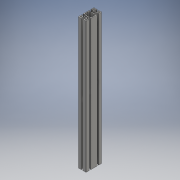
# Autodesk Inventor part: 240614_day3060_500
Saved by Autodesk Inventor 2016 (Build 200138000, 138)
## iProperties
Created: 2024-06-14
Part Number: 240614_day3060_500
Material: 일반
Document SubType Name: Modeling
Designer: pc
Density: 1 g/cm^3
Appearance: 기본값
Author: pc
Autodesk Inventor part; units mm, degrees
ref_plane "YZ Plane" through (0, 0, 0) normal (1, 0, 0) x (0, 1, 0)
ref_plane "XZ Plane" through (0, 0, 0) normal (0, 1, 0) x (-1, 0, 0)
ref_plane "XY Plane" through (0, 0, 0) normal (0, 0, 1) x (1, 0, 0)
sketch "스케치1" plane through (0, 0, 0) normal (0, 0, 1) x (1, 0, 0)
  line L0 (-12.2024, 9.85) -> (-6.681, 9.85)
  arc A0 (-6.681, 9.85) -> (-6.4593, 9.9479) centre (-6.681, 10.15) ccw
  arc A1 (-6.4593, 9.9479) -> (-4.5203, 14.4821) centre (-12.0024, 15) ccw
  line L1 (-4.5203, 14.4821) -> (-4.0024, 15)
  line L2 (-4.0024, 15) -> (-4.5203, 15.5179)
  arc A2 (-4.5203, 15.5179) -> (-6.4593, 20.0521) centre (-12.0024, 15) ccw
  arc A3 (-6.4593, 20.0521) -> (-6.681, 20.15) centre (-6.681, 19.85) ccw
  line L3 (-6.681, 20.15) -> (-12.2024, 20.15)
  arc A4 (-12.2024, 20.15) -> (-12.5024, 19.85) centre (-12.2024, 19.85) ccw
  line L4 (-12.5024, 19.85) -> (-12.5024, 18.45)
  arc A5 (-12.8024, 18.15) -> (-12.5024, 18.45) centre (-12.8024, 18.45) ccw
  line L5 (-12.8024, 18.15) -> (-15.0024, 18.15)
  line L6 (-15.0024, 18.15) -> (-15.0024, 28.9756)
  arc A6 (-14.0024, 29.9756) -> (-15.0024, 28.9756) centre (-14.0024, 28.9756) ccw
  line L7 (-14.0024, 29.9756) -> (-3.1524, 29.9756)
  line L8 (-3.1524, 29.9756) -> (-3.1524, 27.8)
  arc A7 (-3.4524, 27.5) -> (-3.1524, 27.8) centre (-3.4524, 27.8) ccw
  line L9 (-3.4524, 27.5) -> (-4.8524, 27.5)
  arc A8 (-4.8524, 27.5) -> (-5.1524, 27.2) centre (-4.8524, 27.2) ccw
  line L10 (-5.1524, 27.2) -> (-5.1524, 21.6786)
  arc A9 (-5.1524, 21.6786) -> (-5.0545, 21.4569) centre (-4.8524, 21.6786) ccw
  arc A10 (-5.0545, 21.4569) -> (-0.5203, 19.5179) centre (-0.0024, 27) ccw
  line L11 (-0.5203, 19.5179) -> (-0.0024, 19)
  line L12 (-0.0024, 19) -> (0.5155, 19.5179)
  arc A11 (0.5155, 19.5179) -> (5.0497, 21.4569) centre (-0.0024, 27) ccw
  arc A12 (5.0497, 21.4569) -> (5.1476, 21.6786) centre (4.8476, 21.6786) ccw
  line L13 (5.1476, 21.6786) -> (5.1476, 27.2)
  arc A13 (5.1476, 27.2) -> (4.8476, 27.5) centre (4.8476, 27.2) ccw
  line L14 (4.8476, 27.5) -> (3.4476, 27.5)
  arc A14 (3.1476, 27.8) -> (3.4476, 27.5) centre (3.4476, 27.8) ccw
  line L15 (3.1476, 27.8) -> (3.1476, 29.9756)
  line L16 (3.1476, 29.9756) -> (13.9976, 29.9756)
  arc A15 (14.9976, 28.9756) -> (13.9976, 29.9756) centre (13.9976, 28.9756) ccw
  line L17 (14.9976, 28.9756) -> (14.9976, 18.15)
  line L18 (14.9976, 18.15) -> (12.7976, 18.15)
  arc A16 (12.4976, 18.45) -> (12.7976, 18.15) centre (12.7976, 18.45) ccw
  line L19 (12.4976, 18.45) -> (12.4976, 19.85)
  arc A17 (12.4976, 19.85) -> (12.1976, 20.15) centre (12.1976, 19.85) ccw
  line L20 (12.1976, 20.15) -> (6.6762, 20.15)
  arc A18 (6.6762, 20.15) -> (6.4544, 20.0521) centre (6.6762, 19.85) ccw
  arc A19 (6.4544, 20.0521) -> (4.5155, 15.5179) centre (11.9976, 15) ccw
  line L21 (4.5155, 15.5179) -> (3.9976, 15)
  line L22 (3.9976, 15) -> (4.5155, 14.4821)
  arc A20 (4.5155, 14.4821) -> (6.4544, 9.9479) centre (11.9976, 15) ccw
  arc A21 (6.4544, 9.9479) -> (6.6762, 9.85) centre (6.6762, 10.15) ccw
  line L23 (6.6762, 9.85) -> (12.1976, 9.85)
  arc A22 (12.1976, 9.85) -> (12.4976, 10.15) centre (12.1976, 10.15) ccw
  line L24 (12.4976, 10.15) -> (12.4976, 11.55)
  arc A23 (12.7976, 11.85) -> (12.4976, 11.55) centre (12.7976, 11.55) ccw
  line L25 (12.7976, 11.85) -> (14.9976, 11.85)
  line L26 (14.9976, 11.85) -> (14.9976, -11.85)
  line L27 (14.9976, -11.85) -> (12.7976, -11.85)
  arc A24 (12.4976, -11.55) -> (12.7976, -11.85) centre (12.7976, -11.55) ccw
  line L28 (12.4976, -11.55) -> (12.4976, -10.15)
  arc A25 (12.4976, -10.15) -> (12.1976, -9.85) centre (12.1976, -10.15) ccw
  line L29 (12.1976, -9.85) -> (6.6762, -9.85)
  arc A26 (6.6762, -9.85) -> (6.4544, -9.9479) centre (6.6762, -10.15) ccw
  arc A27 (6.4544, -9.9479) -> (4.5155, -14.4821) centre (11.9976, -15) ccw
  line L30 (4.5155, -14.4821) -> (3.9976, -15)
  line L31 (3.9976, -15) -> (4.5155, -15.5179)
  arc A28 (4.5155, -15.5179) -> (6.4544, -20.0521) centre (11.9976, -15) ccw
  arc A29 (6.4544, -20.0521) -> (6.6762, -20.15) centre (6.6762, -19.85) ccw
  line L32 (6.6762, -20.15) -> (12.1976, -20.15)
  arc A30 (12.1976, -20.15) -> (12.4976, -19.85) centre (12.1976, -19.85) ccw
  line L33 (12.4976, -19.85) -> (12.4976, -18.45)
  arc A31 (12.7976, -18.15) -> (12.4976, -18.45) centre (12.7976, -18.45) ccw
  line L34 (12.7976, -18.15) -> (14.9976, -18.15)
  line L35 (14.9976, -18.15) -> (14.9976, -29.0244)
  arc A32 (13.9976, -30.0244) -> (14.9976, -29.0244) centre (13.9976, -29.0244) ccw
  line L36 (13.9976, -30.0244) -> (3.1476, -30.0244)
  line L37 (3.1476, -30.0244) -> (3.1476, -27.8)
  arc A33 (3.4476, -27.5) -> (3.1476, -27.8) centre (3.4476, -27.8) ccw
  line L38 (3.4476, -27.5) -> (4.8476, -27.5)
  arc A34 (4.8476, -27.5) -> (5.1476, -27.2) centre (4.8476, -27.2) ccw
  line L39 (5.1476, -27.2) -> (5.1476, -21.6786)
  arc A35 (5.1476, -21.6786) -> (5.0497, -21.4569) centre (4.8476, -21.6786) ccw
  arc A36 (5.0497, -21.4569) -> (0.5155, -19.5179) centre (-0.0024, -27) ccw
  line L40 (0.5155, -19.5179) -> (-0.0024, -19)
  line L41 (-0.0024, -19) -> (-0.5203, -19.5179)
  arc A37 (-0.5203, -19.5179) -> (-5.0545, -21.4569) centre (-0.0024, -27) ccw
  arc A38 (-5.0545, -21.4569) -> (-5.1524, -21.6786) centre (-4.8524, -21.6786) ccw
  line L42 (-5.1524, -21.6786) -> (-5.1524, -27.2)
  arc A39 (-5.1524, -27.2) -> (-4.8524, -27.5) centre (-4.8524, -27.2) ccw
  line L43 (-4.8524, -27.5) -> (-3.4524, -27.5)
  arc A40 (-3.1524, -27.8) -> (-3.4524, -27.5) centre (-3.4524, -27.8) ccw
  line L44 (-3.1524, -27.8) -> (-3.1524, -30.0244)
  line L45 (-3.1524, -30.0244) -> (-14.0024, -30.0244)
  arc A41 (-15.0024, -29.0244) -> (-14.0024, -30.0244) centre (-14.0024, -29.0244) ccw
  line L46 (-15.0024, -29.0244) -> (-15.0024, -18.15)
  line L47 (-15.0024, -18.15) -> (-12.8024, -18.15)
  arc A42 (-12.5024, -18.45) -> (-12.8024, -18.15) centre (-12.8024, -18.45) ccw
  line L48 (-12.5024, -18.45) -> (-12.5024, -19.85)
  arc A43 (-12.5024, -19.85) -> (-12.2024, -20.15) centre (-12.2024, -19.85) ccw
  line L49 (-12.2024, -20.15) -> (-6.681, -20.15)
  arc A44 (-6.681, -20.15) -> (-6.4593, -20.0521) centre (-6.681, -19.85) ccw
  arc A45 (-6.4593, -20.0521) -> (-4.5203, -15.5179) centre (-12.0024, -15) ccw
  line L50 (-4.5203, -15.5179) -> (-4.0024, -15)
  line L51 (-4.0024, -15) -> (-4.5203, -14.4821)
  arc A46 (-4.5203, -14.4821) -> (-6.4593, -9.9479) centre (-12.0024, -15) ccw
  arc A47 (-6.4593, -9.9479) -> (-6.681, -9.85) centre (-6.681, -10.15) ccw
  line L52 (-6.681, -9.85) -> (-12.2024, -9.85)
  arc A48 (-12.2024, -9.85) -> (-12.5024, -10.15) centre (-12.2024, -10.15) ccw
  line L53 (-12.5024, -10.15) -> (-12.5024, -11.55)
  arc A49 (-12.8024, -11.85) -> (-12.5024, -11.55) centre (-12.8024, -11.55) ccw
  line L54 (-12.8024, -11.85) -> (-15.0024, -11.85)
  line L55 (-15.0024, -11.85) -> (-15.0024, 11.85)
  line L56 (-15.0024, 11.85) -> (-12.8024, 11.85)
  arc A50 (-12.5024, 11.55) -> (-12.8024, 11.85) centre (-12.8024, 11.55) ccw
  line L57 (-12.5024, 11.55) -> (-12.5024, 10.15)
  arc A51 (-12.5024, 10.15) -> (-12.2024, 9.85) centre (-12.2024, 10.15) ccw
  arc A52 (-2.2146, 16.16) -> (-2.2146, 13.84) centre (0, 15) ccw
  line L58 (-2.2146, 13.84) -> (-2.79, 13.2645)
  arc A53 (-2.79, 13.2645) -> (-2.79, 12.8403) centre (-2.5779, 13.0524) ccw
  line L59 (-2.79, 12.8403) -> (-2.1597, 12.21)
  arc A54 (-2.1597, 12.21) -> (-1.7355, 12.21) centre (-1.9476, 12.4221) ccw
  line L60 (-1.7355, 12.21) -> (-1.16, 12.7854)
  arc A55 (-1.16, 12.7854) -> (1.16, 12.7854) centre (0, 15) ccw
  line L61 (1.16, 12.7854) -> (1.7355, 12.21)
  arc A56 (1.7355, 12.21) -> (2.1597, 12.21) centre (1.9476, 12.4221) ccw
  line L62 (2.1597, 12.21) -> (2.79, 12.8403)
  arc A57 (2.79, 12.8403) -> (2.79, 13.2645) centre (2.5779, 13.0524) ccw
  line L63 (2.79, 13.2645) -> (2.2146, 13.84)
  arc A58 (2.2146, 13.84) -> (2.2146, 16.16) centre (0, 15) ccw
  line L64 (2.2146, 16.16) -> (2.79, 16.7355)
  arc A59 (2.79, 16.7355) -> (2.79, 17.1597) centre (2.5779, 16.9476) ccw
  line L65 (2.79, 17.1597) -> (2.1597, 17.79)
  arc A60 (2.1597, 17.79) -> (1.7355, 17.79) centre (1.9476, 17.5779) ccw
  line L66 (1.7355, 17.79) -> (1.16, 17.2146)
  arc A61 (1.16, 17.2146) -> (-1.16, 17.2146) centre (0, 15) ccw
  line L67 (-1.16, 17.2146) -> (-1.7355, 17.79)
  arc A62 (-1.7355, 17.79) -> (-2.1597, 17.79) centre (-1.9476, 17.5779) ccw
  line L68 (-2.1597, 17.79) -> (-2.79, 17.1597)
  arc A63 (-2.79, 17.1597) -> (-2.79, 16.7355) centre (-2.5779, 16.9476) ccw
  line L69 (-2.79, 16.7355) -> (-2.2146, 16.16)
  line L70 (-1.16, -12.7854) -> (-1.7355, -12.21)
  arc A64 (-1.7355, -12.21) -> (-2.1597, -12.21) centre (-1.9476, -12.4221) ccw
  line L71 (-2.1597, -12.21) -> (-2.79, -12.8403)
  arc A65 (-2.79, -12.8403) -> (-2.79, -13.2645) centre (-2.5779, -13.0524) ccw
  line L72 (-2.79, -13.2645) -> (-2.2146, -13.84)
  arc A66 (-2.2146, -13.84) -> (-2.2146, -16.16) centre (0, -15) ccw
  line L73 (-2.2146, -16.16) -> (-2.79, -16.7355)
  arc A67 (-2.79, -16.7355) -> (-2.79, -17.1597) centre (-2.5779, -16.9476) ccw
  line L74 (-2.79, -17.1597) -> (-2.1597, -17.79)
  arc A68 (-2.1597, -17.79) -> (-1.7355, -17.79) centre (-1.9476, -17.5779) ccw
  line L75 (-1.7355, -17.79) -> (-1.16, -17.2146)
  arc A69 (-1.16, -17.2146) -> (1.16, -17.2146) centre (0, -15) ccw
  line L76 (1.16, -17.2146) -> (1.7355, -17.79)
  arc A70 (1.7355, -17.79) -> (2.1597, -17.79) centre (1.9476, -17.5779) ccw
  line L77 (2.1597, -17.79) -> (2.79, -17.1597)
  arc A71 (2.79, -17.1597) -> (2.79, -16.7355) centre (2.5779, -16.9476) ccw
  line L78 (2.79, -16.7355) -> (2.2146, -16.16)
  arc A72 (2.2146, -16.16) -> (2.2146, -13.84) centre (0, -15) ccw
  line L79 (2.2146, -13.84) -> (2.79, -13.2645)
  arc A73 (2.79, -13.2645) -> (2.79, -12.8403) centre (2.5779, -13.0524) ccw
  line L80 (2.79, -12.8403) -> (2.1597, -12.21)
  arc A74 (2.1597, -12.21) -> (1.7355, -12.21) centre (1.9476, -12.4221) ccw
  line L81 (1.7355, -12.21) -> (1.16, -12.7854)
  arc A75 (1.16, -12.7854) -> (-1.16, -12.7854) centre (0, -15) ccw
  circle A76 centre (9.9976, -25.0244) radius 3
  circle A77 centre (9.9976, 24.9756) radius 3
  circle A78 centre (-10.0024, 24.9756) radius 3
  circle A79 centre (-10.0024, -25.0244) radius 3
  arc A80 (-12.5, -4.7272) -> (-9.5038, -7.8454) centre (-9.5023, -4.8454) ccw
  line L82 (-9.5038, -7.8454) -> (-6.1987, -7.847)
  arc A81 (-6.1987, -7.847) -> (6.195, -7.85) centre (0, 0) ccw
  line L83 (6.195, -7.85) -> (9.5, -7.85)
  arc A82 (9.5, -7.85) -> (12.5, -4.85) centre (9.5, -4.85) ccw
  line L84 (12.5, -4.85) -> (12.5, 4.8013)
  arc A83 (12.5, 4.8013) -> (9.5, 7.8013) centre (9.5, 4.8013) ccw
  line L85 (9.5, 7.8013) -> (6.2562, 7.8013)
  arc A84 (6.2562, 7.8013) -> (-6.26, 7.7982) centre (0, 0) ccw
  line L86 (-6.26, 7.7982) -> (-9.5038, 7.7967)
  arc A85 (-9.5038, 7.7967) -> (-12.5, 4.6784) centre (-9.5023, 4.7967) ccw
  line L87 (-12.5, 4.6784) -> (-12.5, -4.7272)
  point P0 (0, 0)
  constraints: 176 end point, 164 point on circle, 86 centre point
extrude "돌출1" add sketch "스케치1" along normal blind 500
